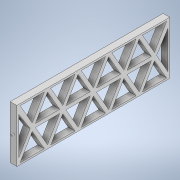
# Autodesk Inventor part: Arm support for middle arms
Saved by Autodesk Inventor 2020.2 (Build 242310000, 310)
## iProperties
Created: 2020-03-31
Part Number: Arm support for middle arms
Material: Generic
Document SubType Name: Modeling
Designer: Amaan Khalid
Density: 1 g/cm^3
Appearance: Default
Author: Amaan Khalid
Autodesk Inventor part; units mm, degrees
ref_plane "YZ Plane" through (0, 0, 0) normal (1, 0, 0) x (0, 1, 0)
ref_plane "XZ Plane" through (0, 0, 0) normal (0, 1, 0) x (-1, 0, 0)
ref_plane "XY Plane" through (0, 0, 0) normal (0, 0, 1) x (1, 0, 0)
sketch "Sketch1" plane through (0, 0, 0) normal (1, 0, 0) x (0, 1, 0)
  line L0 (53.5952, -1.7817) -> (53.5952, -47.6997)
  line L1 (53.5952, -47.6997) -> (93.3614, -24.7407)
  line L2 (93.3614, -24.7407) -> (53.5952, -1.7817)
  line L3 (87.8614, -24.7407) -> (56.3452, -42.9366)
  line L4 (56.3452, -42.9366) -> (56.3452, -6.5449)
  line L5 (56.3452, -6.5449) -> (87.8614, -24.7407)
  line L6 (93.3614, -24.7407) -> (53.5952, -47.6997)
  line L7 (93.3614, -70.6587) -> (53.5952, -47.6997)
  line L8 (93.3614, -24.7407) -> (93.3614, -70.6587)
  line L9 (90.6114, -29.5038) -> (59.0952, -47.6997)
  line L10 (59.0952, -47.6997) -> (90.6114, -65.8956)
  line L11 (90.6114, -65.8956) -> (90.6114, -29.5038)
  line L12 (53.5952, -47.6997) -> (53.5952, -93.6177)
  line L13 (53.5952, -93.6177) -> (93.3614, -70.6587)
  line L14 (56.3452, -88.8546) -> (56.3452, -52.4628)
  line L15 (56.3452, -52.4628) -> (87.8614, -70.6587)
  line L16 (87.8614, -70.6587) -> (56.3452, -88.8546)
  line L17 (93.3614, -70.6587) -> (93.3614, -116.5767)
  line L18 (93.3614, -116.5767) -> (53.5952, -93.6177)
  line L19 (90.6114, -111.8136) -> (90.6114, -75.4218)
  line L20 (59.0952, -93.6177) -> (90.6114, -111.8136)
  line L21 (90.6114, -75.4218) -> (59.0952, -93.6177)
  line L22 (53.5952, -93.6177) -> (53.5952, -139.5357)
  line L23 (56.3452, -134.7726) -> (56.3452, -98.3808)
  line L24 (53.5952, -139.5357) -> (93.3614, -116.5767)
  line L25 (87.8614, -116.5767) -> (56.3452, -134.7726)
  line L26 (56.3452, -98.3808) -> (87.8614, -116.5767)
  line L27 (93.3614, -116.5767) -> (93.3614, -162.4947)
  line L28 (90.6114, -121.3398) -> (59.0952, -139.5357)
  line L29 (59.0952, -139.5357) -> (90.6114, -157.7315)
  line L30 (93.3614, -162.4947) -> (53.5952, -139.5357)
  line L31 (90.6114, -157.7315) -> (90.6114, -121.3398)
  line L32 (53.5952, -139.5357) -> (53.5952, -185.4537)
  line L33 (53.5952, -185.4537) -> (93.3614, -162.4947)
  line L34 (87.8614, -162.4947) -> (56.3452, -180.6905)
  line L35 (56.3452, -180.6905) -> (56.3452, -144.2988)
  line L36 (56.3452, -144.2988) -> (87.8614, -162.4947)
  line L37 (53.5952, -47.6997) -> (13.8291, -24.7407)
  line L38 (13.8291, -24.7407) -> (53.5952, -1.7817)
  line L39 (19.3291, -24.7407) -> (50.8452, -42.9366)
  line L40 (50.8452, -42.9366) -> (50.8452, -6.5449)
  line L41 (50.8452, -6.5449) -> (19.3291, -24.7407)
  line L42 (53.5952, -47.6997) -> (13.8291, -24.7407)
  line L43 (13.8291, -70.6587) -> (53.5952, -47.6997)
  line L44 (13.8291, -24.7407) -> (13.8291, -70.6587)
  line L45 (16.5791, -29.5038) -> (48.0952, -47.6997)
  line L46 (48.0952, -47.6997) -> (16.5791, -65.8956)
  line L47 (16.5791, -65.8956) -> (16.5791, -29.5038)
  line L48 (13.8291, -70.6587) -> (53.5952, -47.6997)
  line L49 (53.5952, -93.6177) -> (13.8291, -70.6587)
  line L50 (50.8452, -52.4628) -> (19.3291, -70.6587)
  line L51 (50.8452, -88.8546) -> (50.8452, -52.4628)
  line L52 (19.3291, -70.6587) -> (50.8452, -88.8546)
  line L53 (13.8291, -116.5767) -> (53.5952, -93.6177)
  line L54 (19.3291, -116.5767) -> (50.8452, -134.7726)
  line L55 (50.8452, -134.7726) -> (50.8452, -98.3808)
  line L56 (53.5952, -139.5357) -> (13.8291, -116.5767)
  line L57 (50.8452, -98.3808) -> (19.3291, -116.5767)
  line L58 (53.5952, -93.6177) -> (13.8291, -70.6587)
  line L59 (16.5791, -75.4218) -> (48.0952, -93.6177)
  line L60 (13.8291, -70.6587) -> (13.8291, -116.5767)
  line L61 (16.5791, -111.8136) -> (16.5791, -75.4218)
  line L62 (13.8291, -116.5767) -> (53.5952, -93.6177)
  line L63 (48.0952, -93.6177) -> (16.5791, -111.8136)
  line L64 (13.8291, -162.4947) -> (53.5952, -139.5357)
  line L65 (50.8452, -180.6905) -> (50.8452, -144.2988)
  line L66 (53.5952, -185.4537) -> (13.8291, -162.4947)
  line L67 (50.8452, -144.2988) -> (19.3291, -162.4947)
  line L68 (19.3291, -162.4947) -> (50.8452, -180.6905)
  line L69 (53.5952, -139.5357) -> (13.8291, -116.5767)
  line L70 (13.8291, -116.5767) -> (13.8291, -162.4947)
  line L71 (16.5791, -157.7315) -> (16.5791, -121.3398)
  line L72 (16.5791, -121.3398) -> (48.0952, -139.5357)
  line L73 (13.8291, -162.4947) -> (53.5952, -139.5357)
  line L74 (48.0952, -139.5357) -> (16.5791, -157.7315)
  line L75 (13.8291, -24.7407) -> (13.8291, 21.1773)
  line L76 (13.8291, 21.1773) -> (53.5952, -1.7817)
  line L77 (93.3614, -24.7407) -> (93.3614, 21.1773)
  line L78 (93.3614, 21.1773) -> (53.5952, -1.7817)
  line L79 (93.3614, 21.1773) -> (13.8291, 21.1773)
  line L80 (93.3614, -162.4947) -> (93.3614, -208.4127)
  line L81 (93.3614, -208.4127) -> (53.5952, -185.4537)
  line L82 (13.8291, -162.4947) -> (13.8291, -208.4127)
  line L83 (13.8291, -208.4127) -> (53.5952, -185.4537)
  line L84 (93.3614, -208.4127) -> (13.8291, -208.4127)
  line L85 (16.5791, -19.9776) -> (16.5791, 16.4141)
  line L86 (48.0952, -1.7817) -> (16.5791, -19.9776)
  line L87 (16.5791, 16.4141) -> (48.0952, -1.7817)
  line L88 (90.6114, -19.9776) -> (90.6114, 16.4141)
  line L89 (90.6114, 16.4141) -> (59.0952, -1.7817)
  line L90 (59.0952, -1.7817) -> (90.6114, -19.9776)
  line L91 (59.0952, -185.4537) -> (90.6114, -203.6495)
  line L92 (90.6114, -203.6495) -> (90.6114, -167.2578)
  line L93 (90.6114, -167.2578) -> (59.0952, -185.4537)
  line L94 (48.0952, -185.4537) -> (16.5791, -203.6495)
  line L95 (16.5791, -203.6495) -> (16.5791, -167.2578)
  line L96 (16.5791, -167.2578) -> (48.0952, -185.4537)
  line L97 (58.0291, 18.4222) -> (80.2383, 18.4222)
  line L98 (80.2383, 18.4222) -> (53.5952, 1.3996)
  line L99 (53.5952, 1.3996) -> (24.1112, 18.4222)
  line L100 (24.1112, 18.4222) -> (58.0291, 18.4222)
  line L101 (58.0291, -205.6576) -> (80.2383, -205.6576)
  line L102 (80.2383, -205.6576) -> (53.5952, -188.635)
  line L103 (53.5952, -188.635) -> (24.1112, -205.6576)
  line L104 (24.1112, -205.6576) -> (58.0291, -205.6576)
  dimension "d13" = 2.75
  constraints: 210 end point, 61 symmetric about line, 5 vertical, 3 collinear, 2 point on line, 1 parallel, 2 other
  measures "d13" distance between parallel lines of L1 L3
extrude "Extrusion1" add sketch "Sketch1" along normal blind 10
sketch "Sketch4" plane through (0, 13.8291, 21.1773) normal (0, 0, 1) x (1, 0, 0)
  line L0 (0, 79.5323) -> (10, 79.5323) projected
  circle A0 centre (5, 39.7661) radius 1.27
  point P0 (0, -13.8291)
  dimension "d41" = 2.54
  constraints: 1 centre point
  measures "d41" diameter of A0
extrude "Extrusion4" add sketch "Sketch4" along normal blind 3
sketch "Sketch5" plane through (0, 13.8291, -208.4127) normal (0, 0, -1) x (-1, 0, 0)
  line L0 (0, 39.7661) -> (-10, 39.7661) projected
  circle A0 centre (-5, 39.7661) radius 1.27
  point P0 (0, -13.8291)
  dimension "d44" = 2.54
  constraints: 1 centre point, 1 midpoint
  measures "d44" diameter of A0
extrude "Extrusion5" add sketch "Sketch5" along normal blind 3
body "Solid1"
